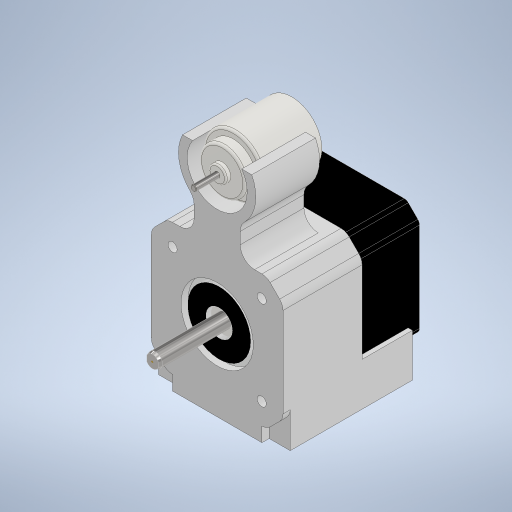
# Autodesk Inventor part: ustepper-generator
Saved by Autodesk Inventor 2024.1 (Build 281209000, 209)
## iProperties
Created: 2026-03-27
Part Number: ustepper-generator
Material: Generic
Document SubType Name: Modeling
Designer: iwheard
Density: 1 g/cm^3
Appearance: Default
Author: iwheard
Autodesk Inventor part; units mm, degrees
ref_plane "YZ Plane" through (0, 0, 0) normal (1, 0, 0) x (0, 1, 0)
ref_plane "XZ Plane" through (0, 0, 0) normal (0, 1, 0) x (-1, 0, 0)
ref_plane "XY Plane" through (0, 0, 0) normal (0, 0, 1) x (1, 0, 0)
sketch "Sketch1" plane through (0, 0, 0) normal (0, 0, 1) x (1, 0, 0)
  line L0 (0, 41.8) -> (41.8, 41.8)
  line L1 (41.8, 41.8) -> (41.8, 0)
  line L2 (41.8, 0) -> (0, 0)
  line L3 (0, 0) -> (0, 41.8)
  dimension "d0" = 41.8
  dimension "d1" = 41.8
  constraints: 8 end point, 1 coincident
  measures "d0" distance between parallel lines of L2 L0
  measures "d1" distance between parallel lines of L1 L3
extrude "Extrusion1" add sketch "Sketch1" against normal blind 47
chamfer "Chamfer1" distance 4.5 angle 45 4 edges at (0, 41.8, -23.5) (41.8, 41.8, -23.5) (41.8, 0, -23.5) (0, 0, -23.5)
fillet "Fillet1" radius 2 8 edges at (4.5, 41.8, -23.5) (37.3, 41.8, -23.5) (41.8, 37.3, -23.5) (41.8, 4.5, -23.5) (0, 37.3, -23.5) (37.3, 0, -23.5) (0, 4.5, -23.5) (4.5, 0, -23.5)
sketch "Sketch2" plane through (0, 0, 0) normal (0, 0, 1) x (1, 0, 0)
  circle A0 centre (20.9, 20.9) radius 11
  line L0 (41.8, 5.3284) -> (41.8, 36.4716) projected
  line L1 (0, 36.4716) -> (0, 5.3284) projected
  line L2 (5.3284, 0) -> (36.4716, 0) projected
  line L3 (36.4716, 41.8) -> (5.3284, 41.8) projected
  circle A1 centre (20.9, 20.9) radius 4.575
  point P0 (0, 0)
  dimension "d8" = 22
  dimension "d9" = 41.8
  dimension "d10" = 41.8
  dimension "d11" = 20.9
  dimension "d12" = 20.9
  dimension "d15" = 9.15
  constraints: 2 centre point, 1 concentric
  measures "d8" diameter of A0
  measures "d9" distance between parallel lines of L0 L1
  measures "d10" distance between parallel lines of L2 L3
  measures "d11" distance from line of L1 A0.centre
  measures "d12" distance from line of L2 A0.centre
  measures "d15" diameter of A1
extrude "Extrusion2" add sketch "Sketch2" along normal blind 1.79
sketch "Sketch3" plane through (20.9, 20.9, 0) normal (0, 0, 1) x (1, 0, 0)
  circle A0 centre (0, 0) radius 2.5
  circle A1 centre (0, 0) radius 4.575 projected
  point P0 (-20.9, -20.9)
  dimension "d16" = 5
  constraints: 1 centre point, 1 concentric
  measures "d16" diameter of A0
extrude "Extrusion3" add sketch "Sketch3" along normal blind 25 contours A0
chamfer "Chamfer2" distance 0.3 distance2 1 1 edges at (18.4, 20.9, 25) measured on face at (18.9, 20.9, 25)
sketch "Sketch4" plane through (20.9, 20.9, 25) normal (0, 0, 1) x (1, 0, 0)
  line L0 (-5.914, 4.6163) -> (-2, 4.6163)
  line L1 (-2, 4.6163) -> (-2, -4.7728)
  line L2 (-2, -4.7728) -> (-5.914, -4.7728)
  line L3 (-5.914, -4.7728) -> (-5.914, 4.6163)
  point P0 (-20.9, -20.9)
  point P1 (0, 0)
  dimension "d22" = 2
  constraints: 8 end point, 1 vertical alignment
  measures "d22" distance from line of point (0, 0) L1
extrude "Extrusion4" cut sketch "Sketch4" against normal blind 15
fillet "Fillet2" radius 1 1 edges at (18.4, 20.9, 10)
sketch "Sketch5" plane through (0, 0, 0) normal (0, 0, 1) x (1, 0, 0)
  circle A0 centre (5.4, 36.4) radius 1.6
  line L0 (36.4716, 41.8) -> (5.3284, 41.8) projected
  line L1 (0, 36.4716) -> (0, 5.3284) projected
  circle A1 centre (36.4, 36.4) radius 1.6
  circle A2 centre (36.4, 5.4) radius 1.6
  circle A3 centre (5.4, 5.4) radius 1.6
  line L2 (41.8, 5.3284) -> (41.8, 36.4716) projected
  line L3 (5.3284, 0) -> (36.4716, 0) projected
  point P0 (0, 0)
  dimension "d26" = 5.4
  dimension "d27" = 5.4
  dimension "d28" = 5.4
  dimension "d29" = 31
  dimension "d30" = 5.4
  dimension "d31" = 3.2
  constraints: 4 centre point, 3 equal radius, 2 horizontal alignment, 2 vertical alignment
  measures "d26" distance from line of A0.centre L0
  measures "d27" distance from line of L1 A0.centre
  measures "d28" distance from line of A1.centre L2
  measures "d29" distance of A1.centre A0.centre
  measures "d30" distance from line of L3 A2.centre
  measures "d31" diameter of A0
extrude "Extrusion5" cut sketch "Sketch5" against normal blind 6
sketch "Sketch6" plane through (0, 0, 0) normal (0, 0, 1) x (1, 0, 0)
  circle A0 centre (5.4, 5.4) radius 1.6 projected
  circle A1 centre (5.4, 36.4) radius 1.6 projected
  circle A2 centre (36.4, 5.4) radius 1.6 projected
  circle A3 centre (36.4, 36.4) radius 1.6 projected
  arc A4 (3.9142, 0.5858) -> (5.3284, 0) centre (5.3284, 2) ccw projected
  line L0 (5.3284, 0) -> (36.4716, 0) projected
  arc A5 (36.4716, 0) -> (37.8858, 0.5858) centre (36.4716, 2) ccw projected
  line L1 (41.2142, 3.9142) -> (37.8858, 0.5858) projected
  arc A6 (41.2142, 3.9142) -> (41.8, 5.3284) centre (39.8, 5.3284) ccw projected
  line L2 (41.8, 5.3284) -> (41.8, 36.4716) projected
  arc A7 (41.8, 36.4716) -> (41.2142, 37.8858) centre (39.8, 36.4716) ccw projected
  line L3 (37.8858, 41.2142) -> (41.2142, 37.8858) projected
  arc A8 (37.8858, 41.2142) -> (36.4716, 41.8) centre (36.4716, 39.8) ccw projected
  line L4 (36.4716, 41.8) -> (5.3284, 41.8) projected
  arc A9 (5.3284, 41.8) -> (3.9142, 41.2142) centre (5.3284, 39.8) ccw projected
  line L5 (0.5858, 37.8858) -> (3.9142, 41.2142) projected
  arc A10 (0.5858, 37.8858) -> (0, 36.4716) centre (2, 36.4716) ccw projected
  line L6 (0, 36.4716) -> (0, 5.3284) projected
  arc A11 (0, 5.3284) -> (0.5858, 3.9142) centre (2, 5.3284) ccw projected
  line L7 (3.9142, 0.5858) -> (0.5858, 3.9142) projected
  circle A12 centre (20.9, 20.9) radius 11 projected
  line L8 (36.4716, -2) -> (5.3284, -2)
  arc A13 (2.5, -0.8284) -> (5.3284, -2) centre (5.3284, 2) ccw
  line L9 (2.5, -0.8284) -> (-0.8284, 2.5)
  arc A14 (-2, 5.3284) -> (-0.8284, 2.5) centre (2, 5.3284) ccw
  line L10 (-2, 5.3284) -> (-2, 36.4716)
  arc A15 (-0.8284, 39.3) -> (-2, 36.4716) centre (2, 36.4716) ccw
  line L11 (-0.8284, 39.3) -> (2.5, 42.6284)
  arc A16 (5.3284, 43.8) -> (2.5, 42.6284) centre (5.3284, 39.8) ccw
  line L12 (5.3284, 43.8) -> (36.4716, 43.8)
  arc A17 (39.3, 42.6284) -> (36.4716, 43.8) centre (36.4716, 39.8) ccw
  line L13 (39.3, 42.6284) -> (42.6284, 39.3)
  arc A18 (43.8, 36.4716) -> (42.6284, 39.3) centre (39.8, 36.4716) ccw
  line L14 (43.8, 36.4716) -> (43.8, 5.3284)
  arc A19 (42.6284, 2.5) -> (43.8, 5.3284) centre (39.8, 5.3284) ccw
  line L15 (42.6284, 2.5) -> (39.3, -0.8284)
  arc A20 (36.4716, -2) -> (39.3, -0.8284) centre (36.4716, 2) ccw
  circle A21 centre (20.9, 20.9) radius 12.5841
  point P0 (0, 0)
  dimension "d34" = 2
  constraints: 16 end point, 16 point on circle, 9 centre point, 15 other
  measures "d34" distance between parallel lines of L8 L0
extrude "Extrusion6" add sketch "Sketch6" along normal blind 2.5 separate body contours L7 A11 L6 A10 L5 A9 L4 A8 L3 A7 L2 A6 L1 A5 L0 A4 | L8 A13 L9 A14 L10 A15 L11 A16 L12 A17 L13 A18 L14 A19 L15 A20
sketch "Sketch7" plane through (0, 0, 0) normal (0, 0, -1) x (-1, 0, 0)
  line L0 (2, 8) -> (-43.8, 8)
  line L1 (-43.8, 8) -> (-43.8, -2)
  line L2 (-43.8, -2) -> (2, -2)
  line L3 (2, -2) -> (2, 8)
  line L4 (-5.3284, -2) -> (-36.4716, -2) projected
  line L5 (-43.8, 5.3284) -> (-43.8, 36.4716) projected
  arc A0 (-43.8, 5.3284) -> (-42.6284, 2.5) centre (-39.8, 5.3284) ccw projected
  line L6 (-39.3, -0.8284) -> (-42.6284, 2.5) projected
  arc A1 (-39.3, -0.8284) -> (-36.4716, -2) centre (-36.4716, 2) ccw projected
  line L7 (-5.3284, -2) -> (-36.4716, -2) projected
  arc A2 (-5.3284, -2) -> (-2.5, -0.8284) centre (-5.3284, 2) ccw projected
  line L8 (0.8284, 2.5) -> (-2.5, -0.8284) projected
  arc A3 (0.8284, 2.5) -> (2, 5.3284) centre (-2, 5.3284) ccw projected
  line L9 (2, 36.4716) -> (2, 5.3284) projected
  arc A4 (2, 36.4716) -> (0.8284, 39.3) centre (-2, 36.4716) ccw projected
  line L10 (-2.5, 42.6284) -> (0.8284, 39.3) projected
  arc A5 (-2.5, 42.6284) -> (-5.3284, 43.8) centre (-5.3284, 39.8) ccw projected
  line L11 (-36.4716, 43.8) -> (-5.3284, 43.8) projected
  arc A6 (-36.4716, 43.8) -> (-39.3, 42.6284) centre (-36.4716, 39.8) ccw projected
  line L12 (-42.6284, 39.3) -> (-39.3, 42.6284) projected
  arc A7 (-42.6284, 39.3) -> (-43.8, 36.4716) centre (-39.8, 36.4716) ccw projected
  circle A8 centre (-5.4, 5.4) radius 1.6 projected
  circle A9 centre (-5.4, 36.4) radius 1.6 projected
  circle A10 centre (-36.4, 5.4) radius 1.6 projected
  circle A11 centre (-36.4, 36.4) radius 1.6 projected
  line L13 (-5.3284, 0) -> (-36.4716, 0) projected
  circle A12 centre (-5.4, 5.4) radius 1.6 projected
  circle A13 centre (-5.4, 36.4) radius 1.6 projected
  circle A14 centre (-36.4, 5.4) radius 1.6 projected
  circle A15 centre (-36.4, 36.4) radius 1.6 projected
  arc A16 (-5.3284, 0) -> (-3.9142, 0.5858) centre (-5.3284, 2) ccw projected
  line L14 (-5.3284, 0) -> (-36.4716, 0) projected
  arc A17 (-37.8858, 0.5858) -> (-36.4716, 0) centre (-36.4716, 2) ccw projected
  line L15 (-41.2142, 3.9142) -> (-37.8858, 0.5858) projected
  arc A18 (-41.8, 5.3284) -> (-41.2142, 3.9142) centre (-39.8, 5.3284) ccw projected
  line L16 (-41.8, 5.3284) -> (-41.8, 36.4716) projected
  arc A19 (-41.2142, 37.8858) -> (-41.8, 36.4716) centre (-39.8, 36.4716) ccw projected
  line L17 (-37.8858, 41.2142) -> (-41.2142, 37.8858) projected
  arc A20 (-36.4716, 41.8) -> (-37.8858, 41.2142) centre (-36.4716, 39.8) ccw projected
  line L18 (-36.4716, 41.8) -> (-5.3284, 41.8) projected
  arc A21 (-3.9142, 41.2142) -> (-5.3284, 41.8) centre (-5.3284, 39.8) ccw projected
  line L19 (-0.5858, 37.8858) -> (-3.9142, 41.2142) projected
  arc A22 (0, 36.4716) -> (-0.5858, 37.8858) centre (-2, 36.4716) ccw projected
  line L20 (0, 36.4716) -> (0, 5.3284) projected
  arc A23 (-0.5858, 3.9142) -> (0, 5.3284) centre (-2, 5.3284) ccw projected
  line L21 (-3.9142, 0.5858) -> (-0.5858, 3.9142) projected
  circle A24 centre (-20.9, 20.9) radius 11 projected
  point P0 (0, 0)
  point P1 (0, 8)
  point P2 (-41.8, 8)
  dimension "d37" = 10
  constraints: 8 end point, 4 vertical alignment, 2 horizontal alignment
  measures "d37" distance between parallel lines of L4 L0
extrude "Extrusion7" add sketch "Sketch7" along normal blind 42.5 contours L3 A3 L8 A2 L2 A1 L6 A0 L1 L0 L16 A18 L15 A17 L13 A16 L21 A23 L20 | L3 L2 A2 L8 A3 | A0 L6 A1 L2 L1 bodies 2
sketch "Sketch8" plane through (-2, -2, 0) normal (0, -1, 0) x (1, 0, 0)
  line L0 (7.3284, 0) -> (0, 0) projected
  line L1 (0, 0) -> (0, -42.5) projected
  line L2 (45.8, -42.5) -> (0, -42.5) projected
  line L3 (45.8, 0) -> (45.8, -42.5) projected
  line L4 (38.4716, 0) -> (38.4716, 2.5) projected
  line L5 (7.3284, 2.5) -> (38.4716, 2.5) projected
  line L6 (7.3284, 0) -> (7.3284, 2.5) projected
  line L7 (7.3284, 0) -> (0, 0) projected
  line L8 (0, 0) -> (0, -42.5) projected
  line L9 (45.8, -42.5) -> (0, -42.5) projected
  line L10 (45.8, 0) -> (45.8, -42.5) projected
  line L11 (45.8, 0) -> (38.4716, 0) projected
  constraints: 1 other
extrude "Extrusion8" add sketch "Sketch8" along normal blind 5 bodies 2
sketch "Sketch9" plane through (0, 0, 0) normal (0, 0, -1) x (-1, 0, 0)
  line L0 (-43.8, 8) -> (-43.8, 36.4716) projected
  line L1 (2, 36.4716) -> (2, 8) projected
  arc A0 (2, 36.4716) -> (0.8284, 39.3) centre (-2, 36.4716) ccw projected
  line L2 (-2.5, 42.6284) -> (0.8284, 39.3) projected
  arc A1 (-2.5, 42.6284) -> (-5.3284, 43.8) centre (-5.3284, 39.8) ccw projected
  line L3 (-36.4716, 43.8) -> (-5.3284, 43.8) projected
  arc A2 (-36.4716, 43.8) -> (-39.3, 42.6284) centre (-36.4716, 39.8) ccw projected
  line L4 (-42.6284, 39.3) -> (-39.3, 42.6284) projected
  arc A3 (-42.6284, 39.3) -> (-43.8, 36.4716) centre (-39.8, 36.4716) ccw projected
  circle A4 centre (-5.4, 5.4) radius 1.6 projected
  circle A5 centre (-5.4, 36.4) radius 1.6 projected
  circle A6 centre (-36.4, 5.4) radius 1.6 projected
  circle A7 centre (-36.4, 36.4) radius 1.6 projected
  circle A8 centre (-20.9, 20.9) radius 12.5841 projected
  circle A9 centre (-5.4, 5.4) radius 1.6 projected
  circle A10 centre (-5.4, 36.4) radius 1.6 projected
  circle A11 centre (-36.4, 5.4) radius 1.6 projected
  circle A12 centre (-36.4, 36.4) radius 1.6 projected
  arc A13 (-5.3284, 0) -> (-3.9142, 0.5858) centre (-5.3284, 2) ccw projected
  line L5 (-5.3284, 0) -> (-36.4716, 0) projected
  arc A14 (-37.8858, 0.5858) -> (-36.4716, 0) centre (-36.4716, 2) ccw projected
  line L6 (-41.2142, 3.9142) -> (-37.8858, 0.5858) projected
  arc A15 (-41.8, 5.3284) -> (-41.2142, 3.9142) centre (-39.8, 5.3284) ccw projected
  line L7 (-41.8, 5.3284) -> (-41.8, 36.4716) projected
  arc A16 (-41.2142, 37.8858) -> (-41.8, 36.4716) centre (-39.8, 36.4716) ccw projected
  line L8 (-37.8858, 41.2142) -> (-41.2142, 37.8858) projected
  arc A17 (-36.4716, 41.8) -> (-37.8858, 41.2142) centre (-36.4716, 39.8) ccw projected
  line L9 (-36.4716, 41.8) -> (-5.3284, 41.8) projected
  arc A18 (-3.9142, 41.2142) -> (-5.3284, 41.8) centre (-5.3284, 39.8) ccw projected
  line L10 (-0.5858, 37.8858) -> (-3.9142, 41.2142) projected
  arc A19 (0, 36.4716) -> (-0.5858, 37.8858) centre (-2, 36.4716) ccw projected
  line L11 (0, 36.4716) -> (0, 5.3284) projected
  arc A20 (-0.5858, 3.9142) -> (0, 5.3284) centre (-2, 5.3284) ccw projected
  line L12 (-3.9142, 0.5858) -> (-0.5858, 3.9142) projected
  circle A21 centre (-20.9, 20.9) radius 11 projected
  line L13 (-5.3284, 42.35) -> (-36.4716, 42.35)
  arc A22 (-36.4716, 42.35) -> (-38.2747, 41.6031) centre (-36.4716, 39.8) ccw
  line L14 (-38.2747, 41.6031) -> (-41.6031, 38.2747)
  arc A23 (-41.6031, 38.2747) -> (-42.35, 36.4716) centre (-39.8, 36.4716) ccw
  line L15 (-42.35, 36.4716) -> (-42.35, 5.3284)
  arc A24 (-42.35, 5.3284) -> (-41.6031, 3.5253) centre (-39.8, 5.3284) ccw
  line L16 (-41.6031, 3.5253) -> (-38.2747, 0.1969)
  arc A25 (-38.2747, 0.1969) -> (-36.4716, -0.55) centre (-36.4716, 2) ccw
  line L17 (-36.4716, -0.55) -> (-5.3284, -0.55)
  arc A26 (-5.3284, -0.55) -> (-3.5253, 0.1969) centre (-5.3284, 2) ccw
  line L18 (-3.5253, 0.1969) -> (-0.1969, 3.5253)
  arc A27 (-0.1969, 3.5253) -> (0.55, 5.3284) centre (-2, 5.3284) ccw
  line L19 (0.55, 5.3284) -> (0.55, 36.4716)
  arc A28 (0.55, 36.4716) -> (-0.1969, 38.2747) centre (-2, 36.4716) ccw
  line L20 (-0.1969, 38.2747) -> (-3.5253, 41.6031)
  arc A29 (-3.5253, 41.6031) -> (-5.3284, 42.35) centre (-5.3284, 39.8) ccw
  line L21 (-43.8, 8) -> (-41.8, 8) projected
  line L22 (-41.8, 8) -> (-41.8, 5.3284) projected
  arc A30 (-41.8, 5.3284) -> (-41.2142, 3.9142) centre (-39.8, 5.3284) ccw projected
  line L23 (-41.2142, 3.9142) -> (-37.8858, 0.5858) projected
  arc A31 (-37.8858, 0.5858) -> (-36.4716, 0) centre (-36.4716, 2) ccw projected
  line L24 (-36.4716, 0) -> (-5.3284, 0) projected
  arc A32 (-5.3284, 0) -> (-3.9142, 0.5858) centre (-5.3284, 2) ccw projected
  line L25 (-3.9142, 0.5858) -> (-0.5858, 3.9142) projected
  arc A33 (-0.5858, 3.9142) -> (0, 5.3284) centre (-2, 5.3284) ccw projected
  line L26 (0, 5.3284) -> (0, 8) projected
  line L27 (0, 8) -> (2, 8) projected
  point P0 (0, 0)
  dimension "d42" = 1.45
  constraints: 16 end point, 16 point on circle, 8 centre point, 15 other
  measures "d42" distance between parallel lines of L13 L3
extrude "Extrusion9" add sketch "Sketch9" along normal blind 25 contours L0 A3 L4 A2 L3 A1 L2 A0 L1 L27 L19 A28 L20 A29 L13 A22 L14 A23 L15 L21 bodies 2
sketch "Sketch18" plane through (0, 0, 2.5) normal (0, 0, 1) x (1, 0, 0)
  circle A0 centre (20.9, 20.9) radius 45
  arc A1 (18.9, 19.9835) -> (18.9, 21.8165) centre (20.9, 20.9) ccw projected
  circle A2 centre (20.9, 65.9) radius 0.98
  point P0 (0, 0)
  dimension "d79" = 90
  dimension "d80" = 1.96
  constraints: 2 vertical alignment, 1 centre point, 3 other
  measures "d80" diameter of A2
extrude "Extrusion16" add sketch "Sketch18" along normal blind 8.27 separate body contours A2 A0 | A0 A2 picked at (20.9391, 65.5749) picked at (20.9377, 66.2237)
fillet "Fillet6" radius 0.2 1 edges at (19.92, 65.9, 10.77)
sketch "Sketch19" plane through (20.9, 65.9, 2.5) normal (0, 0, -1) x (-1, 0, 0)
  circle A0 centre (0, 0) radius 3.015
  circle A1 centre (0, 0) radius 0.98 projected
  point P0 (20.9, -65.9)
  dimension "d84" = 6.03
  constraints: 1 centre point, 1 concentric
  measures "d84" diameter of A0
extrude "Extrusion17" add sketch "Sketch19" along normal blind 1.73 bodies 3
sketch "Sketch20" plane through (20.9, 65.9, 0.77) normal (0, 0, -1) x (-1, 0, 0)
  circle A0 centre (0, 0) radius 8
  circle A1 centre (0, 0) radius 3.015 projected
  point P0 (20.9, -65.9)
  dimension "d87" = 16
  constraints: 1 centre point, 1 concentric
  measures "d87" diameter of A0
extrude "Extrusion18" add sketch "Sketch20" along normal blind 3.84 bodies 3
fillet "Fillet7" radius 0.5 1 edges at (23.915, 65.9, 2.5)
fillet "Fillet8" radius 0.8 1 edges at (28.9, 65.9, 0.77)
sketch "Sketch21" plane through (20.9, 65.9, -3.07) normal (0, 0, -1) x (-1, 0, 0)
  circle A0 centre (0, 0) radius 10.44
  circle A1 centre (0, 0) radius 8 projected
  point P0 (20.9, -65.9)
  dimension "d92" = 20.88
  constraints: 1 centre point, 1 concentric
  measures "d92" diameter of A0
extrude "Extrusion19" add sketch "Sketch21" along normal blind 20.4 contours A0 | A1 bodies 3
fillet "Fillet9" radius 0.8 1 edges at (31.34, 65.9, -3.07)
sketch "Sketch22" plane through (0, 0, 2.5) normal (0, 0, 1) x (1, 0, 0)
  line L0 (43.8, 5.3284) -> (43.8, 36.4716) projected
  arc A0 (43.8, 36.4716) -> (42.6284, 39.3) centre (39.8, 36.4716) ccw projected
  line L1 (42.6284, 39.3) -> (39.3, 42.6284) projected
  arc A1 (39.3, 42.6284) -> (36.4716, 43.8) centre (36.4716, 39.8) ccw projected
  line L2 (36.4716, 43.8) -> (5.3284, 43.8) projected
  arc A2 (5.3284, 43.8) -> (2.5, 42.6284) centre (5.3284, 39.8) ccw projected
  line L3 (2.5, 42.6284) -> (-0.8284, 39.3) projected
  arc A3 (-0.8284, 39.3) -> (-2, 36.4716) centre (2, 36.4716) ccw projected
  line L4 (-2, 36.4716) -> (-2, 5.3284) projected
  arc A4 (-2, 5.3284) -> (-0.8284, 2.5) centre (2, 5.3284) ccw projected
  line L5 (-0.8284, 2.5) -> (2.5, -0.8284) projected
  arc A5 (2.5, -0.8284) -> (5.3284, -2) centre (5.3284, 2) ccw projected
  line L6 (5.3284, -2) -> (5.3284, -7) projected
  line L7 (36.4716, -7) -> (5.3284, -7) projected
  line L8 (36.4716, -2) -> (36.4716, -7) projected
  arc A6 (36.4716, -2) -> (39.3, -0.8284) centre (36.4716, 2) ccw projected
  line L9 (39.3, -0.8284) -> (42.6284, 2.5) projected
  arc A7 (42.6284, 2.5) -> (43.8, 5.3284) centre (39.8, 5.3284) ccw projected
  circle A8 centre (5.4, 5.4) radius 1.6 projected
  circle A9 centre (5.4, 36.4) radius 1.6 projected
  circle A10 centre (36.4, 5.4) radius 1.6 projected
  circle A11 centre (36.4, 36.4) radius 1.6 projected
  circle A12 centre (20.9, 20.9) radius 12.5841 projected
  circle A13 centre (20.9, 65.9) radius 10.44 projected
  circle A14 centre (20.9, 65.9) radius 13.44
  line L10 (4.8804, 83.5656) -> (36.5581, 83.5656)
  line L11 (36.5581, 83.5656) -> (36.5581, 71.9)
  line L12 (36.5581, 71.9) -> (4.5829, 71.9)
  line L13 (4.5829, 71.9) -> (4.8804, 83.5656)
  circle A15 centre (20.9, 65.9) radius 0.78 projected
  line L14 (12.9, 55.1003) -> (28.9, 55.1003)
  line L15 (28.9, 55.1003) -> (28.9, 41.8)
  line L16 (28.9, 41.8) -> (12.9, 41.8)
  line L17 (12.9, 41.8) -> (12.9, 55.1003)
  point P0 (0, 0)
  point P1 (12.9, 43.8)
  point P2 (28.9, 43.8)
  point P3 (32.9264, 71.9)
  point P4 (29.4436, 71.9)
  point P5 (12.3564, 71.9)
  point P6 (8.8736, 71.9)
  dimension "d96" = 3
  dimension "d97" = 6
  dimension "d98" = 8
  dimension "d99" = 8
  constraints: 16 end point, 2 horizontal alignment, 1 vertical alignment, 3 other
  measures "d97" distance from line of L12 A15.centre
  measures "d98" distance from line of L15 A15.centre
  measures "d99" distance from line of A15.centre L17
extrude "Extrusion20" add sketch "Sketch22" against normal blind 22.15 contours L2 L17 A14 L15 | L14 A14 L12 A13 | A14 L14 bodies 2
fillet "Fillet10" radius 5 4 edges at (12.9, 43.8, -8.575) (28.9, 43.8, -8.575) (12.9, 55.1003, -8.575) (28.9, 55.1003, -8.575)
sketch "Sketch23" plane through (0, 0, -42.5) normal (0, 0, -1) x (-1, 0, 0)
  arc A0 (-5.3284, 0) -> (-3.9142, 0.5858) centre (-5.3284, 2) ccw projected
  line L0 (-0.5858, 3.9142) -> (-3.9142, 0.5858) projected
  arc A1 (-0.5858, 3.9142) -> (0, 5.3284) centre (-2, 5.3284) ccw projected
  line L1 (0, 5.3284) -> (0, 36.4716) projected
  arc A2 (0, 36.4716) -> (-0.5858, 37.8858) centre (-2, 36.4716) ccw projected
  line L2 (-3.9142, 41.2142) -> (-0.5858, 37.8858) projected
  arc A3 (-3.9142, 41.2142) -> (-5.3284, 41.8) centre (-5.3284, 39.8) ccw projected
  line L3 (-5.3284, 41.8) -> (-36.4716, 41.8) projected
  arc A4 (-36.4716, 41.8) -> (-37.8858, 41.2142) centre (-36.4716, 39.8) ccw projected
  line L4 (-41.2142, 37.8858) -> (-37.8858, 41.2142) projected
  arc A5 (-41.2142, 37.8858) -> (-41.8, 36.4716) centre (-39.8, 36.4716) ccw projected
  line L5 (-41.8, 36.4716) -> (-41.8, 5.3284) projected
  arc A6 (-41.8, 5.3284) -> (-41.2142, 3.9142) centre (-39.8, 5.3284) ccw projected
  line L6 (-37.8858, 0.5858) -> (-41.2142, 3.9142) projected
  arc A7 (-37.8858, 0.5858) -> (-36.4716, 0) centre (-36.4716, 2) ccw projected
  line L7 (-36.4716, 0) -> (-5.3284, 0) projected
  line L8 (-36.4716, 42.3) -> (-5.3284, 42.3)
  arc A8 (-3.5607, 41.5678) -> (-5.3284, 42.3) centre (-5.3284, 39.8) ccw
  line L9 (-3.5607, 41.5678) -> (-0.2322, 38.2393)
  arc A9 (0.5, 36.4716) -> (-0.2322, 38.2393) centre (-2, 36.4716) ccw
  line L10 (0.5, 36.4716) -> (0.5, 5.3284)
  arc A10 (-0.2322, 3.5607) -> (0.5, 5.3284) centre (-2, 5.3284) ccw
  line L11 (-0.2322, 3.5607) -> (-3.5607, 0.2322)
  arc A11 (-5.3284, -0.5) -> (-3.5607, 0.2322) centre (-5.3284, 2) ccw
  line L12 (-5.3284, -0.5) -> (-36.4716, -0.5)
  arc A12 (-38.2393, 0.2322) -> (-36.4716, -0.5) centre (-36.4716, 2) ccw
  line L13 (-38.2393, 0.2322) -> (-41.5678, 3.5607)
  arc A13 (-42.3, 5.3284) -> (-41.5678, 3.5607) centre (-39.8, 5.3284) ccw
  line L14 (-42.3, 5.3284) -> (-42.3, 36.4716)
  arc A14 (-41.5678, 38.2393) -> (-42.3, 36.4716) centre (-39.8, 36.4716) ccw
  line L15 (-41.5678, 38.2393) -> (-38.2393, 41.5678)
  arc A15 (-36.4716, 42.3) -> (-38.2393, 41.5678) centre (-36.4716, 39.8) ccw
  point P0 (0, 0)
  dimension "d103" = 0.5
  constraints: 16 end point, 16 point on circle, 8 centre point, 15 other
  measures "d103" distance between parallel lines of L3 L8
extrude "Extrusion21" cut sketch "Sketch23" against normal up to surface (42.5 mm away) bodies 2
sketch "Sketch10" plane through (0, 0, 2.5) normal (0, 0, 1) x (1, 0, 0)
  circle A0 centre (20.9, 54.25) radius 10.45
  line L0 (36.4716, 43.8) -> (5.3284, 43.8) projected
  line L1 (-2, 36.4716) -> (-2, 5.3284) projected
  line L2 (43.8, 5.3284) -> (43.8, 36.4716) projected
  point P0 (0, 0)
  dimension "d45" = 20.9
  dimension "d46" = 22.9
  dimension "d47" = 45.8
  constraints: 1 centre point, 1 tangent
  measures "d45" diameter of A0
  measures "d46" distance from line of A0.centre L1
  measures "d47" distance between parallel lines of L2 L1
sketch "Sketch12" plane through (20.9, 54.25, 2.5) normal (0, 0, 1) x (1, 0, 0)
  circle A0 centre (0, 0) radius 8
  circle A1 centre (0, 0) radius 9.698 projected
  point P0 (-20.9, -54.25)
  dimension "d51" = 16
  constraints: 1 centre point, 1 concentric
  measures "d51" diameter of A0
sketch "Sketch13" plane through (20.9, 54.25, 6.3) normal (0, 0, 1) x (1, 0, 0)
  circle A0 centre (0, 0) radius 3.025
  circle A1 centre (0, 0) radius 6.75 projected
  point P0 (-20.9, -54.25)
  dimension "d55" = 6.05
  constraints: 1 centre point, 1 concentric
  measures "d55" diameter of A0
sketch "Sketch14" plane through (20.9, 54.25, 7.8) normal (0, 0, 1) x (1, 0, 0)
  circle A0 centre (0, 0) radius 1
  circle A1 centre (0, 0) radius 3.025 projected
  point P0 (-20.9, -54.25)
  dimension "d58" = 2
  constraints: 1 centre point, 1 concentric
  measures "d58" diameter of A0
sketch "Sketch15" plane through (0, 0, 2.5) normal (0, 0, 1) x (1, 0, 0)
  circle A0 centre (20.9, 54.25) radius 10.45 projected
  line L0 (43.8, 5.3284) -> (43.8, 36.4716) projected
  arc A1 (43.8, 36.4716) -> (42.6284, 39.3) centre (39.8, 36.4716) ccw projected
  line L1 (42.6284, 39.3) -> (39.3, 42.6284) projected
  arc A2 (39.3, 42.6284) -> (36.4716, 43.8) centre (36.4716, 39.8) ccw projected
  line L2 (36.4716, 43.8) -> (5.3284, 43.8) projected
  arc A3 (5.3284, 43.8) -> (2.5, 42.6284) centre (5.3284, 39.8) ccw projected
  line L3 (2.5, 42.6284) -> (-0.8284, 39.3) projected
  arc A4 (-0.8284, 39.3) -> (-2, 36.4716) centre (2, 36.4716) ccw projected
  line L4 (-2, 36.4716) -> (-2, 5.3284) projected
  arc A5 (-2, 5.3284) -> (-0.8284, 2.5) centre (2, 5.3284) ccw projected
  line L5 (-0.8284, 2.5) -> (2.5, -0.8284) projected
  arc A6 (2.5, -0.8284) -> (5.3284, -2) centre (5.3284, 2) ccw projected
  line L6 (5.3284, -2) -> (5.3284, -7) projected
  line L7 (36.4716, -7) -> (5.3284, -7) projected
  line L8 (36.4716, -2) -> (36.4716, -7) projected
  arc A7 (36.4716, -2) -> (39.3, -0.8284) centre (36.4716, 2) ccw projected
  line L9 (39.3, -0.8284) -> (42.6284, 2.5) projected
  arc A8 (42.6284, 2.5) -> (43.8, 5.3284) centre (39.8, 5.3284) ccw projected
  circle A9 centre (5.4, 5.4) radius 1.6 projected
  circle A10 centre (5.4, 36.4) radius 1.6 projected
  circle A11 centre (36.4, 5.4) radius 1.6 projected
  circle A12 centre (36.4, 36.4) radius 1.6 projected
  circle A13 centre (20.9, 20.9) radius 12.5841 projected
  circle A14 centre (20.9, 54.25) radius 12.45
  point P0 (0, 0)
  point P1 (27.6676, 43.8)
  point P2 (14.1324, 43.8)
  point P3 (20.9, 43.8)
  dimension "d62" = 2
  constraints: 1 centre point
  measures "d62" radial gap between concentric circles of A14 A0
sketch "Sketch16" plane through (0, 0, 2.5) normal (0, 0, 1) x (1, 0, 0)
  line L0 (4.7168, 69.7435) -> (41.7479, 69.7435)
  line L1 (41.7479, 69.7435) -> (41.7479, 59.7771)
  line L2 (41.7479, 59.7771) -> (4.7168, 59.7771)
  line L3 (4.7168, 59.7771) -> (4.7168, 69.7435)
  point P0 (0, 0)
  dimension "d70" = 33.35
  dimension "d76" = 33.35
  dimension "d78" = 33.35
  constraints: 2 centre point, 2 concentric, 1 equal radius
equation "\"d1\" = d0"
equation "\"d11\" = 0.5 * d9"
equation "\"d12\" = 0.5 * d10"
equation "\"d26\" = d28"
equation "\"d27\" = d28"
equation "\"d30\" = d28"
equation "\"d99\" = d98"
equation "\"d46\" = 0.5 * d47"
body "Solid7"
